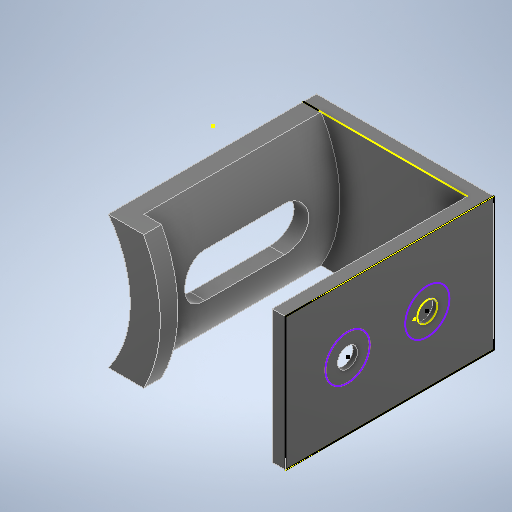
# Autodesk Inventor part: headphones_hook1.1
Saved by Autodesk Inventor 2025.1 (Build 291241000, 241)
## iProperties
Created: 2024-10-23
Part Number: headphones_hook1.1
Material: Generic
Document SubType Name: Modeling
Designer: kamil
Density: 1 g/cm^3
Appearance: Smooth - Black
Author: kamil
Autodesk Inventor part; units mm, degrees
ref_plane "YZ Plane" through (0, 0, 0) normal (1, 0, 0) x (0, 1, 0)
ref_plane "XZ Plane" through (0, 0, 0) normal (0, 1, 0) x (-1, 0, 0)
ref_plane "XY Plane" through (0, 0, 0) normal (0, 0, 1) x (1, 0, 0)
sketch "Sketch1" plane through (0, 0, 0) normal (1, 0, 0) x (0, 1, 0)
  line L0 (-15, -15) -> (15, -15)
  line L1 (15, -15) -> (15, 15)
  line L2 (15, 15) -> (-15, 15)
  line L3 (-15, 15) -> (-15, -15)
  line L4 (-15, -15) -> (15, 15) construction
  line L5 (15, -15) -> (-15, 15) construction
  point P0 (0, 0)
  dimension "d0" = 30
  dimension "d1" = 30
  constraints: 12 end point, 2 midpoint, 2 parallel, 1 horizontal, 1 perpendicular
  measures "d0" distance of L2.end L1.end
  measures "d1" distance of L1.end L0.end
extrude "Extrusion1" add sketch "Sketch1" along normal blind 3
sketch "Sketch2" plane through (0, -15, -15) normal (0, 0, -1) x (-1, 0, 0)
  line L0 (0, 30) -> (-3, 30) projected
  line L1 (-3, 30) -> (37, 30)
  line L2 (37, 30) -> (37, 0)
  line L3 (37, 0) -> (-3, 0)
  line L4 (-3, 0) -> (-3, 30)
  point P0 (0, 15)
  dimension "d4" = 40
  dimension "d5" = 30
  constraints: 8 end point, 2 parallel, 1 horizontal, 1 perpendicular
  measures "d4" distance of L2.end L3.end
  measures "d5" distance of L1.end L2.end
extrude "Extrusion2" add sketch "Sketch2" along normal blind 3
sketch "Sketch3" plane through (0, -15, -15) normal (0, 0, 1) x (1, 0, 0)
  line L0 (0, 0) -> (-37, 0) projected
  line L1 (-37, 0) -> (-37, 30) projected
  arc A0 (-37, 0) -> (-37, 30) centre (-57.325, 15) ccw
  point P0 (0, 15)
  constraints: 2 point on circle, 1 centre point
extrude "Extrusion3" cut sketch "Sketch3" against normal blind 3
sketch "Sketch4" plane through (0, -15, -15) normal (0, 0, 1) x (1, 0, 0)
  line L0 (-37, 30) -> (0, 30) projected
  arc A0 (-37, 0) -> (-37, 30) centre (-57.325, 15) ccw projected
  line L1 (-33.6755, 30) -> (-37, 30)
  point P0 (0, 15)
  constraints: 2 end point, 1 collinear, 1 point on line
sketch "Sketch5" plane through (0, -15, -15) normal (0, 0, 1) x (1, 0, 0)
  arc A0 (-37, 0) -> (-37, 30) centre (-57.325, 15) ccw projected
  line L0 (-37, 30) -> (-33, 30)
  line L1 (-37, 30) -> (0, 30) projected
  line L2 (0, 0) -> (-37, 0) projected
  arc A1 (-33, 0) -> (-33, 30) centre (-57.325, 15) ccw
  line L3 (-33, 0) -> (-37, 0)
  arc A2 (-37, 0) -> (-37, 30) centre (-57.325, 15) ccw
  point P0 (0, 15)
  dimension "d10" = 4
  constraints: 4 end point, 4 point on circle, 2 centre point, 2 concentric, 2 point on line, 1 collinear
  measures "d10" distance of L0.start L0.end
extrude "Extrusion4" add sketch "Sketch5" along normal blind 40
sketch "Sketch6" plane through (0, -15, 25) normal (0, 0, 1) x (1, 0, 0)
  line L0 (-33, 30) -> (-37, 30) projected
  line L1 (-37, 30) -> (-29, 30)
  arc A0 (-37, 0) -> (-37, 30) centre (-57.325, 15) ccw projected
  line L2 (-37, 0) -> (-29, 0)
  arc A1 (-29, 0) -> (-29, 30) centre (-57.325, 15) ccw
  arc A2 (-37, 0) -> (-37, 30) centre (-57.325, 15) ccw
  point P0 (0, 15)
  dimension "d13" = 8
  constraints: 4 end point, 4 point on circle, 2 centre point, 2 concentric, 1 collinear, 1 horizontal
  measures "d13" distance of L0.end L1.end
extrude "Extrusion5" add sketch "Sketch6" along normal blind 4
sketch "Sketch7" plane through (0, -15, 15) normal (0, -1, 0) x (1, 0, 0)
  point P0 (0, -15)
sketch "Sketch8" plane through (0, -15, 15) normal (0, 0, 1) x (1, 0, 0)
  point P0 (0, 15)
sketch "Sketch9" plane through (0, -15, 15) normal (0, -1, 0) x (1, 0, 0)
  line L0 (3, 0) -> (3, -33) projected
  line L1 (3, 0) -> (3, 14)
  line L2 (3, 14) -> (0, 14)
  line L3 (0, 0) -> (3, 0) projected
  line L4 (0, 14) -> (0, 0)
  line L5 (0, 0) -> (3, 0)
  point P0 (0, -15)
  dimension "d16" = 14
  constraints: 8 end point, 2 perpendicular, 1 collinear, 1 vertical
  measures "d16" distance of L0.start L1.end
extrude "Extrusion6" add sketch "Sketch9" against normal blind 30
sketch "Sketch10" plane through (0, 0, 0) normal (-1, 0, 0) x (0, 0, 1)
  point P0 (0, 0)
sketch "Sketch11" plane through (0, 0, 0) normal (-1, 0, 0) x (0, 0, 1)
  arc A0 (14.9299, -5.0174) -> (14.976, 4.9821) centre (15, -0.0179) ccw
  arc A1 (-2.9259, 4.9821) -> (-3, -5.0174) centre (-3, -0.0174) ccw
  line L0 (-15, -15) -> (-15, 15) projected
  line L1 (29, -15) -> (29, 15) projected
  line L2 (14.9299, -5.0174) -> (-3, -5.0174)
  line L3 (15.024, 4.9821) -> (-3.0741, 4.9821)
  line L4 (29, -15) -> (-15, -15) projected
  line L5 (-15, 15) -> (29, 15) projected
  point P0 (0, 0)
  point P1 (-15, 0)
  point P2 (29, 0)
  dimension "d19" = 10
  dimension "d20" = 10
  dimension "d21" = 12
  dimension "d22" = 14
  constraints: 6 point on circle, 4 end point, 3 parallel, 2 centre point, 2 midpoint, 2 point on line, 1 tangent
  measures "d19" diameter of A0
  measures "d20" diameter of A1
  measures "d21" distance of A1.centre point (-15, 0)
  measures "d22" distance of point (29, 0) A0.centre
extrude "Extrusion7" cut sketch "Sketch11" along normal blind 50 contours L2 A1 L3 A0
sketch "Sketch12" plane through (0, 0, 0) normal (-1, 0, 0) x (0, 0, 1)
  circle A0 centre (-3, 0) radius 5
  circle A1 centre (15, 0) radius 5
  line L0 (29, -15) -> (29, 15) projected
  line L1 (-15, -15) -> (-15, 15) projected
  point P0 (0, 0)
  point P1 (29, 0)
  point P2 (-15, 0)
  dimension "d25" = 10
  dimension "d26" = 10
  dimension "d27" = 14
  dimension "d28" = 12
  constraints: 2 centre point, 2 midpoint
  measures "d25" diameter of A0
  measures "d26" diameter of A1
  measures "d27" distance of point (29, 0) A1.centre
  measures "d28" distance of point (-15, 0) A0.centre
extrude "Extrusion8" cut sketch "Sketch12" against normal blind 2
sketch "Sketch13" plane through (2, 0, 15) normal (-1, 0, 0) x (0, 0, 1)
  circle A0 centre (0, 0) radius 2.25
  circle A1 centre (-18, 0) radius 2.25
  circle A2 centre (-18, 0) radius 5 projected
  point P0 (-15, 0)
  dimension "d31" = 4.5
  dimension "d32" = 4.5
  dimension "d33" = 2.75
  constraints: 2 centre point
  measures "d31" diameter of A0
  measures "d32" diameter of A1
  measures "d33" radial gap between concentric circles of A2 A1
extrude "Extrusion9" cut sketch "Sketch13" against normal blind 3 contours A0 | A1
sketch "Sketch14" plane through (3, 0, 0) normal (1, 0, 0) x (0, 0, -1)
  line L0 (-29, 15) -> (18, 15) projected
  line L1 (-29, -15) -> (18, -15) projected
  line L2 (-29, 15) -> (18, 15)
  line L3 (18, 15) -> (18, -15)
  line L4 (18, -15) -> (-29, -15)
  line L5 (-29, -15) -> (-29, 15)
  circle A0 centre (3, 0) radius 2.25 projected
  circle A1 centre (3, 0) radius 5
  circle A2 centre (-15, 0) radius 5 projected
  circle A3 centre (-15, 0) radius 5
  point P0 (0, 0)
  constraints: 8 end point, 2 centre point, 2 coincident, 2 parallel, 1 horizontal, 1 perpendicular
body "Solid1"
